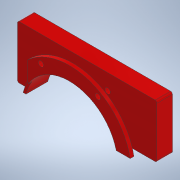
# Autodesk Inventor part: Intake Shroud
Saved by Autodesk Inventor 2022 (Build 260153000, 153)
## iProperties
Created: 2022-10-23
Part Number: Intake Shroud
Material: Generic
Document SubType Name: Modeling
Designer: matt
Density: 1 g/cm^3
Appearance: Default
Author: matt
Autodesk Inventor part; units mm, degrees
ref_plane "YZ Plane" through (0, 0, 0) normal (1, 0, 0) x (0, 1, 0)
ref_plane "XZ Plane" through (0, 0, 0) normal (0, 1, 0) x (-1, 0, 0)
sketch "Sketch1" plane through (0, 0, 0) normal (0, 0, 1) x (1, 0, 0)
  arc A0 (162.0167, 39.368) -> (161.237, 51.1295) centre (107.5651, 41.6649) ccw construction
  line L0 (41.1768, 101.6649) -> (144.3643, 101.6649) construction
  circle A1 centre (63.4018, 101.6649) radius 1.75 construction
  line L1 (63.4018, 133.6649) -> (63.4018, 101.6649) construction
  circle A2 centre (107.4018, 101.6649) radius 1.75 construction
  circle A3 centre (151.4018, 101.6649) radius 1.75 construction
  line L2 (151.4018, 133.6649) -> (151.4018, 101.6649) construction
  circle A4 centre (107.5651, 41.6649) radius 50.5415 construction
  line L3 (52.1155, 51.1295) -> (173.6061, 51.1295) construction
  arc A5 (54.2668, 54.0707) -> (55.4284, 57.5398) centre (-8.1112, 76.8868) ccw
  arc A6 (160.627, 54.1023) -> (55.4284, 57.5398) centre (107.5651, 41.6649) ccw
  arc A7 (57.452, 54.0707) -> (58.2983, 56.666) centre (-8.1112, 76.8868) ccw
  arc A8 (157.5424, 54.0957) -> (58.2983, 56.666) centre (107.5651, 41.6649) ccw
  line L4 (172.3778, 54.1273) -> (157.5424, 54.0957)
  line L5 (57.452, 54.0707) -> (43.812, 54.0707)
  arc A9 (172.3778, 54.1273) -> (42.7416, 54.0707) centre (107.5651, 41.6649) ccw
  circle A10 centre (77.3151, 94.0594) radius 2.8
  line L6 (107.5651, 41.6649) -> (77.3151, 94.0594) construction
  line L7 (107.5651, 41.6649) -> (140.5651, 98.8225) construction
  circle A11 centre (137.8151, 94.0594) radius 2.8
  line L8 (63.1685, 103.3992) -> (63.1685, 99.9305)
  line L9 (63.1685, 90.5007) -> (63.5954, 68.4773)
  line L10 (47.625, 54.0707) -> (47.625, 69.2906)
  line L11 (77.1794, 98.965) -> (81.4957, 96.6297)
  line L12 (81.4957, 96.6297) -> (81.7008, 91.6075)
  line L13 (81.7008, 91.6075) -> (77.4508, 89.1538)
  line L14 (77.4508, 89.1538) -> (73.1346, 91.4891)
  line L15 (73.1346, 91.4891) -> (72.9989, 96.3947)
  line L16 (72.9989, 96.3947) -> (77.1794, 98.965)
  line L17 (137.8151, 89.1519) -> (133.5651, 91.6057)
  line L18 (133.5651, 91.6057) -> (133.5651, 96.5131)
  line L19 (133.5651, 96.5131) -> (137.8151, 98.9669)
  line L20 (137.8151, 98.9669) -> (142.0651, 96.5131)
  line L21 (142.0651, 96.5131) -> (142.0651, 91.6057)
  line L22 (142.0651, 91.6057) -> (137.8151, 89.1519)
  line L23 (41.1685, 300.9746) -> (41.1685, 51.9316)
  line L24 (172.3778, 54.1273) -> (188.3778, 54.1273)
  line L25 (172.3778, 54.1273) -> (188.3778, 54.1273) construction
  line L26 (190.3778, 56.1273) -> (190.3778, 108.8269)
  line L27 (188.3778, 110.8269) -> (43.812, 110.8269)
  line L28 (41.812, 56.0707) -> (41.812, 108.8269)
  arc A12 (41.812, 56.0707) -> (43.812, 54.0707) centre (43.812, 56.0707) ccw
  arc A13 (43.812, 110.8269) -> (41.812, 108.8269) centre (43.812, 108.8269) ccw
  arc A14 (190.3778, 108.8269) -> (188.3778, 110.8269) centre (188.3778, 108.8269) ccw
  arc A15 (188.3778, 54.1273) -> (190.3778, 56.1273) centre (188.3778, 56.1273) ccw
  arc A16 (55.9681, 86.6488) -> (50.5185, 102.1453) centre (50.5185, 93.4388) ccw
  line L29 (50.5185, 102.1453) -> (41.812, 102.1453)
  line L30 (41.812, 75.287) -> (55.9681, 86.6488)
  circle A17 centre (50.5185, 93.4388) radius 4.75
  point P0 (0, 0)
  point P1 (107.4018, 133.6649)
  point P2 (190.3778, 54.1273)
  dimension "d18" = 54.5
  dimension "d21" = 3.5
  dimension "d23" = 3.5
  dimension "d24" = 3.5
  dimension "d28" = 60
  dimension "d29" = 3
  dimension "d30" = 5.6
  dimension "d31" = 60.5
  dimension "d32" = 132
  dimension "d33" = 60
  dimension "d34" = 60
  dimension "d35" = 5.6
  dimension "d36" = 60.5
  dimension "d42" = 54.5
  dimension "d49" = 8.5
  dimension "d50" = 8.5
  dimension "d53" = 18
  dimension "d54" = 0
  dimension "d55" = 2
  constraints: 62 end point, 28 point on circle, 18 centre point, 13 point on line, 11 tangent, 7 perpendicular, 5 coincident, 4 horizontal, 3 equal radius, 1 collinear, 1 vertical, 19 other
  measures "d18" radius of A0
  measures "d21" diameter of A1
  measures "d23" diameter of A2
  measures "d24" diameter of A3
  measures "d28" distance from line of A0.centre L0
  measures "d29" radial gap between concentric circles of A6 A8
  measures "d30" diameter of A10
  measures "d31" distance of A4.centre L6.end
  measures "d32" diameter of A9
  measures "d33" angle of L3 L6
  measures "d34" angle of L7 L6
  measures "d35" diameter of A11
  measures "d36" distance of A0.centre A11.centre
  measures "d42" radius of A6
  measures "d49" distance between parallel lines of L14 L11
  measures "d50" distance between parallel lines of L20 L17
  measures "d53" distance of L4.start point (190.378, 54.127)
  measures "d54" distance between parallel lines of L24 L25
  measures "d55" radius of A12
extrude "Extrusion1" add sketch "Sketch1" along normal blind 4 contours L9 A9 L4 A6 | A6 L4 A8 L9 | L11 L12 L13 L14 L15 L16 | L17 L18 L19 L20 L21 L22
extrude "Extrusion2" add sketch "Sketch1" against normal blind 23 contours A5 A6 L9 A8 A7 L5 | A6 L4 A8 L9
ref_plane "Work Plane1" through (0, 0, -6.55) normal (0, 0, -1) x (-1, 0, 0)
extrude "Extrusion3" add sketch "Sketch1" against normal up to surface (16.45 mm away) from surface at -6.55 contours L5 L10 A9 L9 A6 A5 | L5 A12 A9 L10 | L9 A9 L4 A6 | A9 A12 L28 L30 A16 L29 A13 L27 A14 L26 A15 L24 | L28 L29 A16 L30 | L11 L12 L13 L14 L15 L16 | L17 L18 L19 L20 L21 L22 | A17
extrude "Extrusion5" cut sketch "Sketch1" along normal blind 7 from surface at -23 contours L11 L12 L13 L14 L15 L16 | L17 L18 L19 L20 L21 L22
sketch "Sketch3" plane through (41.812, 56.0707, -23) normal (-1, 0, 0) x (0, 0, 1)
  circle A0 centre (7.5, 13.7262) radius 3 projected
  line L0 (16.45, 22.225) -> (1.5875, 22.225)
  line L1 (1.5875, 22.225) -> (1.5875, 4.7625)
  line L2 (1.5875, 4.7625) -> (16.45, 4.7625)
  line L3 (16.45, 4.7625) -> (16.45, 22.225)
  line L4 (16.45, 52.7561) -> (16.45, 0) projected
  point P0 (23, -56.0707)
  constraints: 8 end point, 2 parallel, 1 collinear, 1 horizontal, 1 perpendicular
extrude "Extrusion6" cut sketch "Sketch3" against normal blind 6 contours A0 | L3 L2 L1 L0
extrude "Extrusion7" cut sketch "Sketch1" against normal blind 4 from surface at -6.55 contours L28 L29 A16 L30 | A17
equation "\"d36\" = d31"
body "Solid1"
